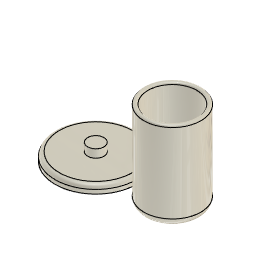
resinCup v1 (Autodesk Fusion 360 design; units mm, degrees)
Autodesk Fusion 360 part; units mm, degrees
sketch "Sketch1" plane through (0, 0, 0) normal (0, 0, 1) x (1, 0, 0)
  circle A0 centre (0, 0) radius 30
  circle A1 centre (0, 0) radius 35
  dimension "d1" = 60
  dimension "d2" = 70
  constraint coincident A0.centre A1.centre
  measures "d1" diameter of A0
  measures "d2" diameter of A1
extrude "Extrude1" add sketch "Sketch1" along normal blind 100 makes body 1
extrude "Extrude2" add sketch "Sketch1" against normal blind 10 contours A0 | A1 bodies 1
fillet "Fillet1" radius 10 1 edges at (-32.6315, 12.6565, -10) on bodies 1
fillet "Fillet2" radius 10 1 edges at (-27.9698, 10.8485, 0) on bodies 1
sketch "Sketch2" plane through (0, 0, -10) normal (0, 0, -1) x (1, 0, 0)
  circle A0 centre (0, 0) radius 25
  circle A1 centre (0, 0) radius 10
  dimension "d11" = 20
  constraint coincident A0.centre A1.centre
  measures "d11" diameter of A1
extrude "Extrude3" cut sketch "Sketch2" against normal blind 45 contours A1 bodies 1
sketch "Sketch3" plane through (0, 0, 0) normal (0, 0, 1) x (1, 0, 0)
  circle A0 centre (-94.3032, 0) radius 50
  circle A1 centre (-94.3032, 0) radius 10
  dimension "d14" = 100
  dimension "d15" = 20
  constraint concentric A0 A1
  measures "d14" diameter of A0
  measures "d15" diameter of A1
extrude "Extrude4" add sketch "Sketch3" against normal blind 10 separate body contours A0 | A1 makes body 2
extrude "Extrude5" add sketch "Sketch3" along normal blind 10 contours A1 bodies 2
fillet "Fillet3" radius 2.5 2 edges at (-32.6315, -12.6565, 100) (-27.9698, 10.8485, 100) on bodies 1
fillet "Fillet4" radius 5 1 edges at (-140.9195, -18.0808, 0) on bodies 2
